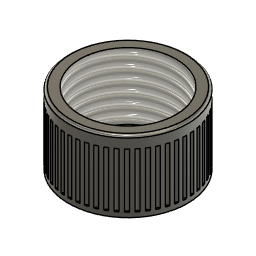
CAP v2 (Autodesk Fusion 360 design; units mm, degrees)
Autodesk Fusion 360 part; units mm, degrees
sketch "Sketch1" plane through (0, 0, 0) normal (0, 1, 0) x (1, 0, 0) in component "Component"
  circle A0 centre (0, 0) radius 2.5
  dimension "d1" = 5
  constraint coincident A0.centre origin
  measures "d1" diameter of A0
sketch "Sketch2" plane through (0, 0, 0) normal (0, 1, 0) x (1, 0, 0) in component "Component"
  circle A0 centre (0, 0) radius 25
  dimension "d4" = 50
  constraint coincident A0.centre origin
  measures "d4" diameter of A0
extrude "Extrude2" add sketch "Sketch2" along normal blind 30 thin wall 1.5 inside in component "Component"
thread "Thread1" "ISO Metric profile 45.0 M45x4.5 6H" major diameter 45.4823 minor diameter 40.4636 pitch 4.5 angle 60 resizes the face on face at (23.3832, 20, 2.3398) in component "Component"
fillet "Fillet1" radius 1 1 edges at (-23.3082, 0, 9.0404) in component "Component"
fillet "Fillet2" radius 1 1 edges at (-23.3082, 30, 9.0404) in component "Component"
sketch "Sketch3" plane through (0, 0, 0) normal (0, 1, 0) x (1, 0, 0) in component "Component"
  circle A0 centre (0.5, -25) radius 0.75
  dimension "d13" = 1.5
  measures "d13" diameter of A0
extrude "Extrude3" cut sketch "Sketch3" along normal blind 25 in component "Component"
pattern_circular "C-Pattern1" count 50 over 360 about axis through (0, 1, 0) along (0, 1, 0) of "Extrude3" in component "Component"
extrude "Extrude4" add sketch "Sketch2" along normal blind 2 in component "Component"
component "Component" placed x (1, 0, 0) y (0, 1, 0) z (0, 0, 1) at (0, 0, 0)
